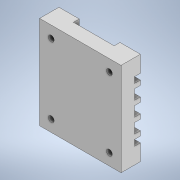
# Autodesk Inventor part: Belt Clamp
Saved by Autodesk Inventor 2020 (Build 240168000, 168)
## iProperties
Created: 2020-03-18
Part Number: Belt Clamp
Material: Generic
Document SubType Name: Modeling
Designer: DasNick
Density: 1 g/cm^3
Appearance: Default
Author: DasNick
Autodesk Inventor part; units mm, degrees
ref_plane "YZ Plane" through (0, 0, 0) normal (1, 0, 0) x (0, 1, 0)
ref_plane "XZ Plane" through (0, 0, 0) normal (0, 1, 0) x (-1, 0, 0)
sketch "Sketch1" plane through (0, 0, 0) normal (0, 0, 1) x (1, 0, 0)
  circle A0 centre (22.3624, 26.3473) radius 1.5875
  circle A1 centre (22.3624, -11.7527) radius 1.5875
  circle A2 centre (-9.3876, 26.3473) radius 1.5875
  circle A3 centre (-9.3876, -11.7527) radius 1.5875
  line L0 (28.7124, 32.6973) -> (-15.7376, 32.6973)
  line L1 (-15.7376, 32.6973) -> (-15.7376, -18.1027)
  line L2 (-15.7376, -18.1027) -> (28.7124, -18.1027)
  line L3 (28.7124, -18.1027) -> (28.7124, 32.6973)
  point P0 (-3.5123, 7.2973)
  dimension "d26" = 50.8
  dimension "d27" = 44.45
  dimension "d28" = 6.35
  dimension "d29" = 6.35
  dimension "d30" = 6.35
  dimension "d31" = 6.35
  dimension "d32" = 6.35
  dimension "d33" = 6.35
  dimension "d34" = 6.35
  dimension "d35" = 6.35
  dimension "d44" = 3.175
  dimension "d45" = 3.175
  dimension "d46" = 3.175
  dimension "d47" = 3.175
  constraints: 8 end point, 4 centre point
  measures "d26" distance of L0.end L1.end
  measures "d27" distance of L0.start L0.end
  measures "d28" distance from line of L1 A3.centre
  measures "d29" distance from line of L2 A3.centre
  measures "d30" distance from line of L2 A1.centre
  measures "d31" distance from line of L3 A1.centre
  measures "d32" distance from line of L0 A0.centre
  measures "d33" distance from line of L0 A2.centre
  measures "d34" distance from line of L1 A2.centre
  measures "d35" distance from line of L3 A0.centre
  measures "d44" diameter of A2
  measures "d45" diameter of A0
  measures "d46" diameter of A1
  measures "d47" diameter of A3
extrude "Extrusion1" add sketch "Sketch1" along normal blind 12.7
sketch "Sketch2" plane through (-15.7376, -18.1027, 0) normal (0, -1, 0) x (1, 0, 0)
  line L0 (11.1075, 69.4178) -> (11.1075, 0)
  line L1 (33.3375, 69.1638) -> (33.3375, 0)
  line L2 (11.1075, 0) -> (33.3375, 0)
  line L3 (0, 9.525) -> (44.45, 9.525)
  line L4 (11.1075, 0) -> (33.3375, 0)
  line L5 (33.3375, 0) -> (33.3375, 5.334)
  line L6 (33.3375, 5.334) -> (11.1075, 5.334)
  line L7 (11.1075, 5.334) -> (11.1075, 0)
  line L8 (0, 0) -> (44.45, 0) projected
  point P0 (15.875, 0)
  point P1 (11.1075, 5.334)
  dimension "d2" = 5.334
  dimension "d21" = 0
  constraints: 16 end point, 1 point on line
  measures "d2" distance of L5.end L4.end
  measures "d21" distance between parallel lines of L8 L2
extrude "Extrusion2" cut sketch "Sketch2" against normal blind 76.2 contours L6 L1 L2 L0
ref_plane "Work Plane1" through (-16.0653, -32.8267, -33.655) normal (0, 0, -1) x (0, 1, 0)
sketch "Sketch3" plane through (17.5999, -18.1027, 5.334) normal (0, 0, -1) x (-1, 0, 0)
  line L0 (0, 0) -> (0, 50.8) projected
  line L1 (0, 36.068) -> (22.23, 36.068)
  line L2 (22.23, 36.068) -> (22.23, 38.608)
  line L3 (22.23, 38.608) -> (0, 38.608)
  line L4 (0, 38.608) -> (0, 36.068)
  line L5 (0, 50.8) -> (22.23, 50.8) projected
  line L6 (33.3375, 65.3946) -> (33.3375, 0) projected
  line L7 (0, 28.068) -> (22.23, 28.068)
  line L8 (22.23, 28.068) -> (22.23, 30.608)
  line L9 (22.23, 30.608) -> (0, 30.608)
  line L10 (0, 30.608) -> (0, 28.068)
  line L11 (0, 20.068) -> (22.23, 20.068)
  line L12 (22.23, 20.068) -> (22.23, 22.608)
  line L13 (22.23, 22.608) -> (0, 22.608)
  line L14 (0, 22.608) -> (0, 20.068)
  line L15 (0, 12.068) -> (22.23, 12.068)
  line L16 (22.23, 12.068) -> (22.23, 14.608)
  line L17 (22.23, 14.608) -> (0, 14.608)
  line L18 (0, 14.608) -> (0, 12.068)
  point P0 (17.5999, 18.1027)
  point P1 (0, 14.608)
  point P2 (0, 12.068)
  point P3 (0, 22.608)
  point P4 (0, 20.068)
  point P5 (0, 30.608)
  point P6 (0, 28.068)
  point P7 (0, 38.608)
  dimension "d6" = 12.192
  dimension "d7" = 2.54
  dimension "d10" = 8
  constraints: 32 end point, 2 parallel, 1 horizontal, 1 perpendicular, 1 point on line, 1 vertical, 24 other
  measures "d6" distance between parallel lines of L5 L3
  measures "d7" distance between parallel lines of L3 L1
  measures "d10" distance of L1.start L7.start
extrude "Extrusion3" add sketch "Sketch3" along normal blind 5.334
sketch "Sketch4" plane through (0, 0, 0) normal (0, 0, -1) x (-1, 0, 0)
  line L0 (-17.5999, 12.5053) -> (4.6301, 12.5053) projected
  line L1 (4.6301, 12.5053) -> (4.6301, 17.9653)
  line L2 (4.6301, 17.9653) -> (-17.5999, 17.9653) projected
  line L3 (-17.5999, 12.5053) -> (-17.5999, 17.9653)
  line L4 (-17.5999, 4.5053) -> (4.6301, 4.5053) projected
  line L5 (4.6301, 4.5053) -> (4.6301, 9.9653)
  line L6 (4.6301, 9.9653) -> (-17.5999, 9.9653) projected
  line L7 (-17.5999, 4.5053) -> (-17.5999, 9.9653)
  line L8 (4.6301, 1.9653) -> (-17.5999, 1.9653) projected
  line L9 (-17.5999, -3.4947) -> (-17.5999, 1.9653)
  line L10 (-17.5999, -3.4947) -> (4.6301, -3.4947) projected
  line L11 (4.6301, -3.4947) -> (4.6301, 1.9653)
  line L12 (4.6301, 20.5053) -> (4.6301, 32.6973) projected
  line L13 (4.6301, 20.5053) -> (20.4326, 20.5053)
  line L14 (20.4326, 20.5053) -> (20.4326, 23.6803)
  line L15 (20.4326, 23.6803) -> (4.6301, 23.6803)
  line L16 (4.6301, 23.6803) -> (4.6301, 20.5053)
  line L17 (4.6301, -6.0347) -> (-17.5999, -6.0347) projected
  line L18 (4.6301, -6.0347) -> (18.5436, -6.0347)
  line L19 (18.5436, -6.0347) -> (18.5436, -9.2097)
  line L20 (18.5436, -9.2097) -> (4.6301, -9.2097)
  line L21 (4.6301, -9.2097) -> (4.6301, -6.0347)
  line L22 (4.6301, 12.5053) -> (4.6301, 17.9653) projected
  line L23 (4.6301, 17.9653) -> (23.203, 17.9653)
  line L24 (23.203, 17.9653) -> (23.203, 12.5053)
  line L25 (23.203, 12.5053) -> (4.6301, 12.5053)
  line L26 (4.6301, 12.5053) -> (4.6301, 17.9653)
  line L27 (4.6301, 9.9653) -> (4.6301, 4.5053) projected
  line L28 (4.6301, 9.9653) -> (22.3845, 9.9653)
  line L29 (22.3845, 9.9653) -> (22.3845, 4.5053)
  line L30 (22.3845, 4.5053) -> (4.6301, 4.5053)
  line L31 (4.6301, 4.5053) -> (4.6301, 9.9653)
  line L32 (4.6301, 1.9653) -> (4.6301, -3.4947) projected
  line L33 (4.6301, 1.9653) -> (21.9437, 1.9653)
  line L34 (21.9437, 1.9653) -> (21.9437, -3.4947)
  line L35 (21.9437, -3.4947) -> (4.6301, -3.4947)
  line L36 (4.6301, -3.4947) -> (4.6301, 1.9653)
  line L37 (-17.5999, 17.9653) -> (-33.0876, 17.9653)
  line L38 (-33.0876, 17.9653) -> (-33.0876, 12.5053)
  line L39 (-33.0876, 12.5053) -> (-17.5999, 12.5053)
  line L40 (-17.5999, 12.5053) -> (-17.5999, 17.9653)
  line L41 (-17.5999, 9.9653) -> (-34.7876, 9.9653)
  line L42 (-34.7876, 9.9653) -> (-34.7876, 4.5053)
  line L43 (-34.7876, 4.5053) -> (-17.5999, 4.5053)
  line L44 (-17.5999, 4.5053) -> (-17.5999, 9.9653)
  line L45 (-17.5999, 1.9653) -> (4.6301, 1.9653) projected
  line L46 (-17.5999, 1.9653) -> (-33.0876, 1.9653)
  line L47 (-33.0876, 1.9653) -> (-33.0876, -3.4947)
  line L48 (-33.0876, -3.4947) -> (-17.5999, -3.4947)
  line L49 (-17.5999, -3.4947) -> (-17.5999, 1.9653)
  line L50 (-17.5999, 20.5053) -> (-30.1912, 20.5053)
  line L51 (-30.1912, 20.5053) -> (-30.1912, 23.6803)
  line L52 (-30.1912, 23.6803) -> (-17.5999, 23.6803)
  line L53 (-17.5999, 23.6803) -> (-17.5999, 20.5053)
  line L54 (-17.5999, -6.0347) -> (-30.1912, -6.0347)
  line L55 (-30.1912, -6.0347) -> (-30.1912, -9.2097)
  line L56 (-30.1912, -9.2097) -> (-17.5999, -9.2097)
  line L57 (-17.5999, -9.2097) -> (-17.5999, -6.0347)
  point P0 (-17.5999, -3.4947)
  point P1 (4.6301, -3.4947)
  point P2 (-17.5999, 4.5053)
  point P3 (4.6301, 4.5053)
  point P4 (-17.5999, 12.5053)
  point P5 (4.6301, 12.5053)
  point P6 (4.6301, 23.6803)
  dimension "d40" = 3.175
  dimension "d41" = 3.175
  dimension "d42" = 3.175
  dimension "d43" = 3.175
  constraints: 92 end point, 20 parallel, 10 horizontal, 10 perpendicular, 4 point on line
  measures "d40" distance of L14.end L13.end
  measures "d41" distance of L18.end L19.end
  measures "d42" distance of L50.end L51.end
  measures "d43" distance of L55.end L54.end
extrude "Extrusion4" cut sketch "Sketch4" against normal blind 5.334 contours L39 L38 L37 L3 | L1 L23 L24 L25 | L43 L42 L41 L7 | L5 L28 L29 L30 | L33 L34 L35 L11 | L9 L48 L47 L46 | L12 L15 L14 L13 | L57 L56 L55 L54 | L18 L19 L20 L21 | L50 L51 L52 L53
sketch "Sketch5" plane through (0, 0, 0) normal (0, 0, -1) x (-1, 0, 0)
  line L0 (17.6982, 39.5282) -> (-30.6897, 39.5282)
  line L1 (-30.6897, 39.5282) -> (-30.6897, -19.7169)
  line L2 (-30.6897, -19.7169) -> (17.6982, -19.7169)
  line L3 (17.6982, -19.7169) -> (17.6982, 39.5282)
  constraints: 8 end point, 2 parallel, 1 horizontal, 1 perpendicular
extrude "Extrusion5" cut sketch "Sketch5" against normal blind 2.159
body "Solid1"
